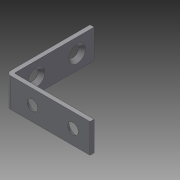
# Autodesk Inventor part: L-Bracket
Saved by Autodesk Inventor 2015 (Build 190159000, 159)
## iProperties
Created: 2017-03-05
Part Number: L-Bracket
Material: Generic
Document SubType Name: Modeling
Designer: 1esh9
Density: 1 g/cm^3
Appearance: Default
Author: 1esh9
Autodesk Inventor part; units mm, degrees
ref_plane "YZ Plane" through (0, 0, 0) normal (1, 0, 0) x (0, 1, 0)
ref_plane "XZ Plane" through (0, 0, 0) normal (0, 1, 0) x (-1, 0, 0)
ref_plane "XY Plane" through (0, 0, 0) normal (0, 0, 1) x (1, 0, 0)
sketch "Sketch1" plane through (0, 0, 0) normal (0, 0, 1) x (1, 0, 0)
  line L0 (0, 38) -> (1.85, 38)
  line L1 (1.85, 38) -> (1.85, 2.35)
  line L2 (0, 38) -> (0, 2)
  line L3 (38, 0) -> (38, 1.85)
  line L4 (38, 1.85) -> (2.35, 1.85)
  line L5 (38, 0) -> (2, 0)
  arc A0 (1.85, 2.35) -> (2.35, 1.85) centre (2.35, 2.35) ccw
  arc A1 (0, 2) -> (2, 0) centre (2, 2) ccw
  point P0 (0, 0)
  dimension "d0" = 1.85
  dimension "d1" = 1.85
  dimension "d2" = 38
  dimension "d3" = 38
  dimension "d4" = 0.5
  dimension "d5" = 2
  constraints: 12 end point, 4 point on circle, 4 tangent, 2 centre point, 2 horizontal, 2 perpendicular, 2 vertical
  measures "d0" distance of L0.start L0.end
  measures "d1" distance of L3.start L3.end
  measures "d2" distance from line of point (0, 0) L3
  measures "d3" distance from line of point (0, 0) L0
  measures "d4" radius of A0
  measures "d5" radius of A1
extrude "Extrusion1" add sketch "Sketch1" along normal blind 13.2
sketch "Sketch2" plane through (1.85, 2.35, 0) normal (1, 0, 0) x (0, 0, -1)
  circle A0 centre (-6.6, 27.975) radius 2.425
  circle A1 centre (-6.6, 9.575) radius 2.425
  line L0 (0, 35.65) -> (-13.2, 35.65) projected
  line L1 (-13.2, 0) -> (-13.2, 35.65) projected
  point P0 (0, -2.35)
  dimension "d8" = 18.4
  dimension "d9" = 4.85
  dimension "d10" = 4.85
  dimension "d11" = 5.25
  dimension "d12" = 13.2
  dimension "d13" = 6.6
  dimension "d14" = 6.6
  constraints: 2 centre point
  measures "d8" distance of A1.centre A0.centre
  measures "d9" diameter of A0
  measures "d10" diameter of A1
  measures "d11" distance edge to line of A0 L0
  measures "d12" distance of L0.start L0.end
  measures "d13" distance from line of L1 A0.centre
  measures "d14" distance from line of L1 A1.centre
sketch "Sketch3" plane through (2.35, 1.85, 0) normal (0, 1, 0) x (1, 0, 0)
  circle A0 centre (27.975, -6.6) radius 2.425
  circle A1 centre (9.575, -6.6) radius 2.425
  line L0 (35.65, -13.2) -> (0, -13.2) projected
  line L1 (35.65, 0) -> (35.65, -13.2) projected
  point P0 (-2.35, 0)
  dimension "d15" = 18.4
  dimension "d16" = 6.6
  dimension "d17" = 6.6
  dimension "d18" = 4.85
  dimension "d19" = 4.85
  dimension "d20" = 5.25
  constraints: 2 centre point
  measures "d15" distance of A1.centre A0.centre
  measures "d16" distance from line of L0 A0.centre
  measures "d17" distance from line of L0 A1.centre
  measures "d18" diameter of A0
  measures "d19" diameter of A1
  measures "d20" distance edge to line of A0 L1
extrude "Extrusion2" cut sketch "Sketch2" against normal blind 13.2
extrude "Extrusion3" cut sketch "Sketch3" against normal blind 13.2
chamfer "Chamfer1" distance 1.4 distance2 1.8 1 edges at (1.85, 30.325, 9.025) measured on face at (1.85, 23.3649, 1.4152)
chamfer "Chamfer2" distance 1.4 distance2 1.8 1 edges at (9.5, 1.85, 6.6) measured on face at (17.5224, 1.85, 1.3976)
chamfer "Chamfer3" distance 1.4 distance2 1.8 1 edges at (1.85, 11.925, 9.025) measured on face at (1.85, 23.2532, 12.238)
chamfer "Chamfer4" distance 1.4 distance2 1.8 1 edges at (27.9, 1.85, 6.6) measured on face at (17.5787, 1.85, 0.9343)
equation "\"d13\" = 0.5 * d12"
equation "\"d14\" = d13"
equation "\"d17\" = d16"
body "Solid1"
